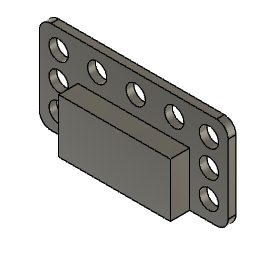
soap holder bracket v2 (Autodesk Fusion 360 design; units mm, degrees)
Autodesk Fusion 360 part; units mm, degrees
sketch "Sketch1" plane through (0, 0, 0) normal (0, 1, 0) x (1, 0, 0)
  line L0 (0, 0) -> (49, 0)
  line L1 (49, 0) -> (49, -24)
  line L2 (49, -24) -> (0, -24)
  line L3 (0, -24) -> (0, 0)
  constraint horizontal L0
  constraint vertical L1
  constraint horizontal L2
  constraint vertical L3
  constraint coincident L0.start L3.end
extrude "Extrude1" add sketch "Sketch1" along normal blind 2
sketch "Sketch2" plane through (0, 0, 0) normal (0, 1, 0) x (1, 0, 0)
  line L0 (10, 0) -> (39, 0)
  line L1 (39, 0) -> (39, -14)
  line L2 (39, -14) -> (10, -14)
  line L3 (10, -14) -> (10, 0)
  constraint horizontal L0
  constraint vertical L1
  constraint horizontal L2
  constraint vertical L3
extrude "Extrude2" add sketch "Sketch2" against normal blind 5
fillet "Fillet1" radius 3 1 edges at (0, 1, 24)
fillet "Fillet2" radius 3 1 edges at (49, 1, 24)
fillet "Fillet3" radius 3 1 edges at (49, 1, 0)
fillet "Fillet4" radius 3 1 edges at (0, 1, 0)
sketch "Sketch3" plane through (0, 0, 0) normal (0, 1, 0) x (1, 0, 0)
  circle A0 centre (5, -5) radius 2.5
  dimension "d13" = 5
  measures "d13" diameter of A0
extrude "Extrude3" cut sketch "Sketch3" along normal blind 3
sketch "Sketch4" plane through (0, 0, 0) normal (0, 1, 0) x (1, 0, 0)
  circle A0 centre (44, -5) radius 2.5
  dimension "d16" = 5
  measures "d16" diameter of A0
extrude "Extrude4" cut sketch "Sketch4" along normal blind 3
sketch "Sketch5" plane through (0, 0, 0) normal (0, 1, 0) x (1, 0, 0)
  circle A0 centre (5, -19) radius 2.5
  dimension "d19" = 5
  measures "d19" diameter of A0
extrude "Extrude5" cut sketch "Sketch5" along normal blind 3
sketch "Sketch6" plane through (0, 0, 0) normal (0, 1, 0) x (1, 0, 0)
  circle A0 centre (44, -19) radius 2.5
  dimension "d22" = 5
  measures "d22" diameter of A0
extrude "Extrude6" cut sketch "Sketch6" along normal blind 3
sketch "Sketch7" plane through (0, 0, 0) normal (0, 1, 0) x (1, 0, 0)
  circle A0 centre (44, -12) radius 2.5
  dimension "d25" = 5
  measures "d25" diameter of A0
extrude "Extrude7" cut sketch "Sketch7" along normal blind 2
sketch "Sketch8" plane through (0, 0, 0) normal (0, 1, 0) x (1, 0, 0)
  circle A0 centre (5, -12) radius 2.5
  dimension "d28" = 5
  measures "d28" diameter of A0
extrude "Extrude8" cut sketch "Sketch8" along normal blind 3
sketch "Sketch9" plane through (0, 0, 0) normal (0, 1, 0) x (1, 0, 0)
  circle A0 centre (25, -19) radius 2.5
  dimension "d31" = 5
  measures "d31" diameter of A0
extrude "Extrude9" cut sketch "Sketch9" along normal blind 3
sketch "Sketch10" plane through (0, 0, 0) normal (0, 1, 0) x (1, 0, 0)
  circle A0 centre (15, -19) radius 2.5
  dimension "d34" = 5
  measures "d34" diameter of A0
extrude "Extrude10" cut sketch "Sketch10" along normal blind 2
sketch "Sketch11" plane through (0, 0, 0) normal (0, 1, 0) x (1, 0, 0)
  circle A0 centre (35, -19) radius 2.5
  dimension "d37" = 5
  measures "d37" diameter of A0
extrude "Extrude11" cut sketch "Sketch11" along normal blind 5
